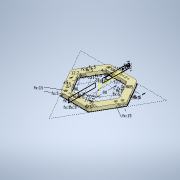
# Autodesk Inventor part: upper_board_mount
Saved by Autodesk Inventor 2021 (Build 250183000, 183)
## iProperties
Created: 2021-01-25
Part Number: upper_board_mount
Material: PC/ABS 플라스틱
Document SubType Name: Modeling
Designer: leejun
Density: 0.357273 g/cm^3
Appearance: 매끄러움 - 물푸레나무색
Author: leejun
Autodesk Inventor part; units mm, degrees
ref_plane "YZ Plane" through (0, 0, 0) normal (1, 0, 0) x (0, 1, 0)
ref_plane "XZ Plane" through (0, 0, 0) normal (0, 1, 0) x (-1, 0, 0)
ref_plane "XY Plane" through (0, 0, 0) normal (0, 0, 1) x (1, 0, 0)
sketch "스케치1" plane through (0, 0, 0) normal (0, 1, 0) x (-1, 0, 0)
  line L0 (128.6603, -74.282) -> (42.8868, -74.282) construction
  line L1 (-128.6603, -74.282) -> (0, 148.5641) construction
  line L2 (0, 148.5641) -> (128.6603, -74.282) construction
  line L3 (40, -69.282) -> (-40, -69.282) construction
  line L4 (-40, -69.282) -> (-40, -56.582) construction
  line L5 (-40, -56.582) -> (40, -56.582) construction
  line L6 (40, -56.582) -> (40, -69.282) construction
  line L7 (-80, 0) -> (-40, 69.282) construction
  line L8 (-40, 69.282) -> (-29.0015, 62.932) construction
  line L9 (-29.0015, 62.932) -> (-69.0015, -6.35) construction
  line L10 (-69.0015, -6.35) -> (-80, 0) construction
  line L11 (40, 69.282) -> (29.0015, 62.932) construction
  line L12 (29.0015, 62.932) -> (69.0015, -6.35) construction
  line L13 (69.0015, -6.35) -> (80, 0) construction
  line L14 (80, 0) -> (40, 69.282) construction
  line L15 (85.7735, 0) -> (42.8868, -74.282) construction
  line L16 (-42.8868, -74.282) -> (-85.7735, 0) construction
  line L17 (42.8868, 74.282) -> (-42.8868, 74.282) construction
  circle A0 centre (72.0007, 1.1551) radius 6.35 construction
  circle A1 centre (64.5007, 14.1455) radius 6.35 construction
  circle A2 centre (-35, -62.932) radius 6.35 construction
  circle A3 centre (-20, -62.932) radius 6.35 construction
  circle A4 centre (-37.0007, 61.7769) radius 6.35 construction
  circle A5 centre (-44.5007, 48.7865) radius 6.35 construction
  circle A6 centre (72.0007, 1.1551) radius 2.65 construction
  circle A7 centre (64.5007, 14.1455) radius 2.65 construction
  circle A8 centre (-20, -62.932) radius 2.65 construction
  circle A9 centre (-35, -62.932) radius 2.65 construction
  circle A10 centre (-44.5007, 48.7865) radius 2.65 construction
  circle A11 centre (-37.0007, 61.7769) radius 2.65 construction
  line L18 (40, -56.582) -> (-40, -69.282) construction
  line L19 (-40, -56.582) -> (40, -69.282) construction
  line L20 (69.0015, -6.35) -> (40, 69.282) construction
  line L21 (80, 0) -> (29.0015, 62.932) construction
  line L22 (-29.0015, 62.932) -> (-80, 0) construction
  line L23 (-69.0015, -6.35) -> (-40, 69.282) construction
  line L24 (72.0007, 1.1551) -> (64.5007, 14.1455) construction
  line L25 (-20, -62.932) -> (-35, -62.932) construction
  line L26 (-37.0007, 61.7769) -> (-44.5007, 48.7865) construction
  circle A12 centre (35, -62.932) radius 2.15
  circle A13 centre (20, -62.932) radius 2.15
  circle A14 centre (44.5007, 48.7865) radius 2.15
  circle A15 centre (37.0007, 61.7769) radius 2.15
  circle A16 centre (-72.0007, 1.1551) radius 2.15
  circle A17 centre (-64.5007, 14.1455) radius 2.15
  line L27 (42.8868, -74.282) -> (-42.8868, -74.282) construction
  line L28 (-42.8868, -74.282) -> (-128.6603, -74.282) construction
  line L29 (0, -62.932) -> (-54.5007, 31.466) construction
  line L30 (-54.5007, 31.466) -> (54.5007, 31.466) construction
  line L31 (54.5007, 31.466) -> (0, -62.932) construction
  line L32 (68.844, -27.6227) -> (58.344, -45.8093) construction
  line L33 (58.344, -45.8093) -> (40.1575, -35.3093) construction
  line L34 (40.1575, -35.3093) -> (50.6575, -17.1227) construction
  line L35 (50.6575, -17.1227) -> (68.844, -27.6227) construction
  line L36 (10.5, 73.432) -> (-10.5, 73.432) construction
  line L37 (-10.5, 73.432) -> (-10.5, 52.432) construction
  line L38 (-10.5, 52.432) -> (10.5, 52.432) construction
  line L39 (10.5, 52.432) -> (10.5, 73.432) construction
  line L40 (-58.344, -45.8093) -> (-68.844, -27.6227) construction
  line L41 (-68.844, -27.6227) -> (-50.6575, -17.1227) construction
  line L42 (-50.6575, -17.1227) -> (-40.1575, -35.3093) construction
  line L43 (-40.1575, -35.3093) -> (-58.344, -45.8093) construction
  line L44 (45.4075, -26.216) -> (-45.4075, -26.216) construction
  line L45 (-45.4075, -26.216) -> (0, 52.432) construction
  line L46 (0, 52.432) -> (45.4075, -26.216) construction
  line L47 (61.8712, 0) -> (30.9356, -53.582)
  line L48 (30.9356, -53.582) -> (-30.9356, -53.582)
  line L49 (-30.9356, -53.582) -> (-61.8712, 0)
  line L50 (-61.8712, 0) -> (-30.9356, 53.582)
  line L51 (-30.9356, 53.582) -> (30.9356, 53.582)
  line L52 (30.9356, 53.582) -> (61.8712, 0)
  line L53 (83.4641, 0) -> (41.7321, -72.282)
  line L54 (41.7321, -72.282) -> (-41.7321, -72.282)
  line L55 (-41.7321, -72.282) -> (-83.4641, 0)
  line L56 (-83.4641, 0) -> (-41.7321, 72.282)
  line L57 (-41.7321, 72.282) -> (41.7321, 72.282)
  line L58 (41.7321, 72.282) -> (83.4641, 0)
  line L59 (68.844, -27.6227) -> (40.1575, -35.3093) construction
  line L60 (58.344, -45.8093) -> (50.6575, -17.1227) construction
  circle A18 centre (54.5007, -31.466) radius 9.35 construction
  line L61 (71.0668, -21.4727) -> (73.9536, -26.4727) construction
  line L62 (73.9536, -26.4727) -> (59.9029, -50.8093) construction
  line L63 (59.9029, -50.8093) -> (54.1293, -50.8093) construction
  line L64 (54.8721, -12.1227) -> (49.0986, -12.1227) construction
  line L65 (49.0986, -12.1227) -> (35.0479, -36.4593) construction
  line L66 (35.0479, -36.4593) -> (37.9347, -41.4593) construction
  line L67 (16.9375, 53.582) -> (14.0507, 48.582) construction
  line L68 (14.0507, 48.582) -> (-14.0507, 48.582) construction
  line L69 (-14.0507, 48.582) -> (-16.9375, 53.582) construction
  line L70 (16.9375, 72.282) -> (14.0507, 77.282) construction
  line L71 (14.0507, 77.282) -> (-14.0507, 77.282) construction
  line L72 (-14.0507, 77.282) -> (-16.9375, 72.282) construction
  line L73 (-37.9347, -41.4593) -> (-35.0479, -36.4593) construction
  line L74 (-35.0479, -36.4593) -> (-49.0986, -12.1227) construction
  line L75 (-49.0986, -12.1227) -> (-54.8721, -12.1227) construction
  line L76 (-71.0668, -21.4727) -> (-73.9536, -26.4727) construction
  line L77 (-73.9536, -26.4727) -> (-59.9029, -50.8093) construction
  line L78 (-59.9029, -50.8093) -> (-54.1293, -50.8093) construction
  line L79 (42.8868, 74.282) -> (40, 69.282) construction
  line L80 (80, 0) -> (85.7735, 0) construction
  line L81 (0, 40) -> (-12.7, 40) construction
  line L82 (-12.7, 40) -> (-12.7, 52.7) construction
  line L83 (-12.7, 52.7) -> (0, 52.7) construction
  line L84 (0, 52.7) -> (0, 40) construction
  line L85 (12.7, -40) -> (0, -40) construction
  line L86 (0, -52.7) -> (12.7, -52.7) construction
  line L87 (12.7, -52.7) -> (12.7, -40) construction
  line L88 (12.7, -52.7) -> (-12.7, 52.7) construction
  line L89 (0, -40) -> (0, -52.7) construction
  line L90 (0, 52.7) -> (0, -52.7) construction
  line L91 (-12.7, 40) -> (-22.7, 40)
  line L92 (-22.7, 40) -> (-22.7, 53.582)
  line L93 (-22.7, 53.582) -> (-12.7, 53.582)
  line L94 (-12.7, 53.582) -> (-12.7, 40)
  line L95 (12.7, -40) -> (22.7, -40)
  line L96 (22.7, -40) -> (22.7, -53.582)
  line L97 (22.7, -53.582) -> (12.7, -53.582)
  line L98 (12.7, -53.582) -> (12.7, -40)
  line L99 (-12.7, 52.7) -> (-22.7, 52.7)
  line L100 (12.7, -52.7) -> (22.7, -52.7)
  point P0 (0, 0)
  point P1 (0, 0)
  point P2 (0, 0)
  point P3 (0, 0)
  point P4 (0, 0)
  point P5 (0, 0)
  point P6 (0, 0)
  dimension "d1" = 12.7
  dimension "d12" = 80
  dimension "d13" = 5.3
  dimension "d14" = 5
  dimension "d15" = 20
  dimension "d16" = 5
  dimension "d17" = 20
  dimension "d18" = 5
  dimension "d19" = 20
  dimension "d79" = 4.3
  dimension "d80" = 5
  dimension "d81" = 15
  dimension "d82" = 5
  dimension "d83" = 15
  dimension "d84" = 5
  dimension "d85" = 15
  dimension "d86" = 5
  dimension "d88" = 21
  dimension "d89" = 3
  dimension "d90" = 3
  dimension "d92" = 5
  dimension "d93" = 5
  dimension "d95" = 5
  dimension "d96" = 5
  dimension "d97" = 5
  dimension "d98" = 5
  dimension "d99" = 5
  dimension "d100" = 5
  dimension "d101" = 5
  dimension "d102" = 5
  dimension "d103" = 5
  dimension "d104" = 5
  dimension "d105" = 5
  dimension "d106" = 5
  dimension "d107" = 5
  dimension "d108" = 5
  dimension "d136" = 5
  dimension "d137" = 5
  dimension "d140" = 12.7
  dimension "d142" = 80
  dimension "d143" = 10
  constraints: 202 end point, 48 parallel, 28 point on line, 19 centre point, 16 equal length, 15 horizontal, 14 tangent, 12 coincident, 11 perpendicular, 10 equal radius, 9 midpoint, 2 collinear, 47 other
  measures "d1" distance of L12.end L13.end
  measures "d12" distance of L11.end L12.end
  measures "d13" diameter of A6
  measures "d14" distance from line of L13 A0.centre
  measures "d15" distance from line of A1.centre L13
  measures "d16" distance from line of L4 A2.centre
  measures "d17" distance from line of L4 A3.centre
  measures "d18" distance from line of L8 A4.centre
  measures "d19" distance from line of L8 A5.centre
  measures "d79" diameter of A12
  measures "d80" distance from line of A12.centre L6
  measures "d81" distance of A13.centre A12.centre
  measures "d82" distance from line of L11 A15.centre
  measures "d83" distance of A15.centre A14.centre
  measures "d84" distance from line of A16.centre L10
  measures "d85" distance of A17.centre A16.centre
  measures "d86" distance between parallel lines of L14 L2
  measures "d88" distance of L33.end L34.end
  measures "d89" distance between parallel lines of L14 L58
  measures "d90" distance between parallel lines of L12 L52
  measures "d92" distance from line of L32.start L61
  measures "d93" distance from line of L63 L32.end
  measures "d95" distance from line of L66 L33.end
  measures "d96" distance from line of L64 L34.end
  measures "d97" distance between parallel lines of L71 L57
  measures "d98" distance from line of L36.start L70
  measures "d99" distance from line of L72 L36.end
  measures "d100" distance between parallel lines of L51 L68
  measures "d101" distance from line of L38.end L67
  measures "d102" distance from line of L37.end L69
  measures "d103" distance between parallel lines of L49 L74
  measures "d104" distance from line of L42.end L73
  measures "d105" distance from line of L75 L41.end
  measures "d106" distance between parallel lines of L77 L55
  measures "d107" distance from line of L40.start L78
  measures "d108" distance from line of L76 L40.end
  measures "d136" distance between parallel lines of L53 L62
  measures "d137" distance between parallel lines of L65 L47
  measures "d140" distance of L85.end L86.start
  measures "d142" distance between parallel lines of L81 L85
  measures "d143" distance of L81.end L91.end
extrude "돌출18" add sketch "스케치1" along normal blind 10
sketch "스케치15" plane through (0, 0, 0) normal (0, -1, 0) x (1, 0, 0)
  line L0 (-41.7321, 72.282) -> (41.7321, 72.282) projected
  line L1 (-83.4641, 0) -> (-41.7321, 72.282) projected
  line L2 (-41.7321, -72.282) -> (-83.4641, 0) projected
  line L3 (41.7321, -72.282) -> (-41.7321, -72.282) projected
  line L4 (83.4641, 0) -> (41.7321, -72.282) projected
  line L5 (41.7321, 72.282) -> (83.4641, 0) projected
  circle A0 centre (-35, -62.932) radius 2.15 projected
  circle A1 centre (-20, -62.932) radius 2.15 projected
  circle A2 centre (-37.0007, 61.7769) radius 2.15 projected
  circle A3 centre (64.5007, 14.1455) radius 2.15 projected
  circle A4 centre (72.0007, 1.1551) radius 2.15 projected
  circle A5 centre (-44.5007, 48.7865) radius 2.15 projected
  line L6 (-61.8712, 0) -> (-30.9356, -53.582) projected
  line L7 (-30.9356, 53.582) -> (-61.8712, 0) projected
  line L8 (30.9356, 53.582) -> (-30.9356, 53.582) projected
  line L9 (61.8712, 0) -> (30.9356, 53.582) projected
  line L10 (30.9356, -53.582) -> (61.8712, 0) projected
  line L11 (-30.9356, -53.582) -> (30.9356, -53.582) projected
  line L12 (-44.5007, 48.7865) -> (-37.0007, 61.7769) construction
  line L13 (-40.1706, 46.2865) -> (-32.6706, 59.2769)
  line L14 (-41.3309, 64.2769) -> (-48.8309, 51.2865)
  arc A6 (-48.8309, 51.2865) -> (-40.1706, 46.2865) centre (-44.5007, 48.7865) ccw
  arc A7 (-32.6706, 59.2769) -> (-41.3309, 64.2769) centre (-37.0007, 61.7769) ccw
  line L15 (-35, -62.932) -> (-20, -62.932) construction
  line L16 (-35, -67.932) -> (-20, -67.932)
  line L17 (-20, -57.932) -> (-35, -57.932)
  arc A8 (-35, -57.932) -> (-35, -67.932) centre (-35, -62.932) ccw
  arc A9 (-20, -67.932) -> (-20, -57.932) centre (-20, -62.932) ccw
  circle A10 centre (72.0007, 1.1551) radius 2.15 projected
  circle A11 centre (64.5007, 14.1455) radius 2.15 projected
  line L18 (72.0007, 1.1551) -> (64.5007, 14.1455) construction
  line L19 (76.3309, 3.6551) -> (68.8309, 16.6455)
  line L20 (60.1706, 11.6455) -> (67.6706, -1.3449)
  arc A12 (67.6706, -1.3449) -> (76.3309, 3.6551) centre (72.0007, 1.1551) ccw
  arc A13 (68.8309, 16.6455) -> (60.1706, 11.6455) centre (64.5007, 14.1455) ccw
  point P0 (0, 0)
  point P1 (-40.7507, 55.2817)
  point P2 (-27.5, -62.932)
  point P3 (68.2507, 7.6503)
  dimension "d148" = 5
  constraints: 24 end point, 12 point on circle, 12 tangent, 6 centre point, 3 midpoint, 3 parallel, 2 equal radius, 1 horizontal
  measures "d148" radius of A6
extrude "돌출20" add sketch "스케치15" along normal blind 5 contours A6 L14 A7 L13 | A8 L17 A9 L16 | A12 L20 A13 L19
fillet "모깎기4" radius 10 12 edges at (41.7321, 5, 72.282) (83.4641, 5, 0) (41.7321, 5, -72.282) (-41.7321, 5, -72.282) (-83.4641, 5, 0) (-41.7321, 5, 72.282) (-61.8712, 5, 0) (-30.9356, 5, 53.582) (30.9356, 5, 53.582) (61.8712, 5, 0) (30.9356, 5, -53.582) (-30.9356, 5, -53.582)
fillet "모깎기4" radius 3 12 edges at (62.0007, 0, 18.4756) (72.5809, 0, 10.1503) (74.5007, 0, -3.175) (63.9206, 0, 5.1503) (-47.0007, 0, 44.4564) (-45.0809, 0, 57.7817) (-34.5007, 0, 66.107) (-36.4206, 0, 52.7817) (-27.5, 0, -57.932) (-15, 0, -62.932) (-27.5, 0, -67.932) (-40, 0, -62.932)
sketch "스케치18" plane through (0, 10, 0) normal (0, 1, 0) x (1, 0, 0)
  arc A0 (-44.6188, -67.282) -> (-35.9585, -72.282) centre (-35.9585, -62.282) ccw projected
  line L0 (-35.9585, -72.282) -> (35.9585, -72.282) projected
  arc A1 (35.9585, -72.282) -> (44.6188, -67.282) centre (35.9585, -62.282) ccw projected
  line L1 (44.6188, -67.282) -> (80.5774, -5) projected
  arc A2 (80.5774, -5) -> (80.5774, 5) centre (71.9171, 0) ccw projected
  line L2 (80.5774, 5) -> (44.6188, 67.282) projected
  arc A3 (44.6188, 67.282) -> (35.9585, 72.282) centre (35.9585, 62.282) ccw projected
  line L3 (35.9585, 72.282) -> (-35.9585, 72.282) projected
  arc A4 (-35.9585, 72.282) -> (-44.6188, 67.282) centre (-35.9585, 62.282) ccw projected
  line L4 (-44.6188, 67.282) -> (-80.5774, 5) projected
  arc A5 (-80.5774, 5) -> (-80.5774, -5) centre (-71.9171, 0) ccw projected
  line L5 (-80.5774, -5) -> (-44.6188, -67.282) projected
  circle A6 centre (-35, 62.932) radius 2.15 projected
  circle A7 centre (-20, 62.932) radius 2.15 projected
  circle A8 centre (-37.0007, -61.7769) radius 2.15 projected
  circle A9 centre (64.5007, -14.1455) radius 2.15 projected
  circle A10 centre (72.0007, -1.1551) radius 2.15 projected
  circle A11 centre (-44.5007, -48.7865) radius 2.15 projected
  line L6 (-58.9845, 5) -> (-33.8224, 48.582) projected
  arc A12 (-25.1621, 53.582) -> (-33.8224, 48.582) centre (-25.1621, 43.582) ccw projected
  line L7 (-25.1621, 53.582) -> (25.1621, 53.582) projected
  arc A13 (33.8224, 48.582) -> (25.1621, 53.582) centre (25.1621, 43.582) ccw projected
  line L8 (33.8224, 48.582) -> (58.9845, 5) projected
  arc A14 (58.9845, -5) -> (58.9845, 5) centre (50.3242, 0) ccw projected
  line L9 (58.9845, -5) -> (33.8224, -48.582) projected
  arc A15 (25.1621, -53.582) -> (33.8224, -48.582) centre (25.1621, -43.582) ccw projected
  line L10 (25.1621, -53.582) -> (-25.1621, -53.582) projected
  arc A16 (-33.8224, -48.582) -> (-25.1621, -53.582) centre (-25.1621, -43.582) ccw projected
  line L11 (-33.8224, -48.582) -> (-58.9845, -5) projected
  arc A17 (-58.9845, 5) -> (-58.9845, -5) centre (-50.3242, 0) ccw projected
  circle A18 centre (-35, 62.932) radius 3.9
  circle A19 centre (-20, 62.932) radius 3.9
  point P0 (0, 0)
  dimension "d167" = 7.8
  constraints: 2 centre point, 2 coincident, 1 equal radius
  measures "d167" diameter of A18
extrude "돌출23" cut sketch "스케치18" against normal blind 3 contours A18 | A19
pattern_circular "원형 패턴5" count 3 over 360 about axis through (0, -10, 0) along (0, 1, 0) of "돌출23"
sketch "스케치25" plane through (0, 0, 0) normal (1, 0, 0) x (0, 1, 0)
  line L0 (12, -91) -> (24.7, -91)
  line L1 (24.7, -91) -> (24.7, -11)
  line L2 (24.7, -11) -> (12, -11)
  line L3 (12, -11) -> (12, -91)
  line L4 (12, 11) -> (24.7, 11)
  line L5 (24.7, 11) -> (24.7, 91)
  line L6 (24.7, 91) -> (12, 91)
  line L7 (12, 91) -> (12, 11)
  line L8 (-4.94, 0) -> (29.64, 0) projected
  line L9 (10, -67.282) -> (10, -5) projected
  circle A0 centre (18.35, -86) radius 6.35
  circle A1 centre (18.35, -86) radius 2.6
  circle A2 centre (18.35, -71) radius 2.6
  point P0 (0, 0)
  dimension "d210" = 12.7
  dimension "d211" = 80
  dimension "d212" = 22
  dimension "d213" = 2
  dimension "d214" = 5
  dimension "d215" = 15
  dimension "d216" = 5.2
  constraints: 16 end point, 4 parallel, 3 centre point, 2 equal length, 2 horizontal, 2 perpendicular, 2 tangent, 1 coincident, 1 collinear, 1 equal radius, 1 vertical alignment, 1 other
  measures "d210" distance of L1.end L2.end
  measures "d211" distance of L0.end L1.end
  measures "d212" distance between parallel lines of L4 L2
  measures "d213" distance between parallel lines of L9 L3
  measures "d214" distance from line of L0 A1.centre
  measures "d215" distance of A2.centre A1.centre
  measures "d216" diameter of A1
sketch "스케치26" plane through (0, 10, 0) normal (0, 1, 0) x (1, 0, 0)
  circle A0 centre (64.5007, -14.1455) radius 3.9 projected
  circle A1 centre (72.0007, -1.1551) radius 3.9 projected
  circle A2 centre (-44.5007, -48.7865) radius 3.9 projected
  circle A3 centre (-37.0007, -61.7769) radius 3.9 projected
  circle A4 centre (-20, 62.932) radius 3.9 projected
  circle A5 centre (-35, 62.932) radius 3.9 projected
  arc A6 (-44.6188, -67.282) -> (-35.9585, -72.282) centre (-35.9585, -62.282) ccw projected
  line L0 (-35.9585, -72.282) -> (35.9585, -72.282) projected
  arc A7 (35.9585, -72.282) -> (44.6188, -67.282) centre (35.9585, -62.282) ccw projected
  line L1 (44.6188, -67.282) -> (80.5774, -5) projected
  arc A8 (80.5774, -5) -> (80.5774, 5) centre (71.9171, 0) ccw projected
  line L2 (80.5774, 5) -> (44.6188, 67.282) projected
  arc A9 (44.6188, 67.282) -> (35.9585, 72.282) centre (35.9585, 62.282) ccw projected
  line L3 (35.9585, 72.282) -> (-35.9585, 72.282) projected
  arc A10 (-35.9585, 72.282) -> (-44.6188, 67.282) centre (-35.9585, 62.282) ccw projected
  line L4 (-44.6188, 67.282) -> (-80.5774, 5) projected
  arc A11 (-80.5774, 5) -> (-80.5774, -5) centre (-71.9171, 0) ccw projected
  line L5 (-80.5774, -5) -> (-44.6188, -67.282) projected
  line L6 (-58.9845, 5) -> (-33.8224, 48.582) projected
  arc A12 (-25.1621, 53.582) -> (-33.8224, 48.582) centre (-25.1621, 43.582) ccw projected
  line L7 (-25.1621, 53.582) -> (25.1621, 53.582) projected
  arc A13 (33.8224, 48.582) -> (25.1621, 53.582) centre (25.1621, 43.582) ccw projected
  line L8 (33.8224, 48.582) -> (58.9845, 5) projected
  arc A14 (58.9845, -5) -> (58.9845, 5) centre (50.3242, 0) ccw projected
  line L9 (58.9845, -5) -> (33.8224, -48.582) projected
  arc A15 (25.1621, -53.582) -> (33.8224, -48.582) centre (25.1621, -43.582) ccw projected
  line L10 (25.1621, -53.582) -> (-25.1621, -53.582) projected
  arc A16 (-33.8224, -48.582) -> (-25.1621, -53.582) centre (-25.1621, -43.582) ccw projected
  line L11 (-33.8224, -48.582) -> (-58.9845, -5) projected
  arc A17 (-58.9845, 5) -> (-58.9845, -5) centre (-50.3242, 0) ccw projected
  line L12 (-25.1621, 53.582) -> (25.1621, 53.582) projected
  line L13 (35.9585, 72.282) -> (-35.9585, 72.282) projected
  line L14 (25.1621, 53.582) -> (0, 53.582)
  line L15 (0, 53.582) -> (0, 72.282)
  line L16 (0, 72.282) -> (25.1621, 72.282)
  line L17 (25.1621, -53.582) -> (-25.1621, -53.582) projected
  line L18 (-35.9585, -72.282) -> (35.9585, -72.282) projected
  line L19 (0, -53.582) -> (-25.1621, -53.582)
  line L20 (-25.1621, -72.282) -> (0, -72.282)
  line L21 (0, -72.282) -> (0, -53.582)
  circle A18 centre (25, 62.932) radius 2.1
  circle A19 centre (10, 62.932) radius 2.1
  circle A20 centre (25, 62.932) radius 9.35 construction
  circle A21 centre (-25, -62.932) radius 2.1
  circle A22 centre (-10, -62.932) radius 2.1
  circle A23 centre (-25, -62.932) radius 9.35 construction
  line L22 (0, 129.02) -> (0, -127.67) projected
  point P0 (0, 0)
  dimension "d217" = 4.2
  dimension "d225" = 15
  dimension "d226" = 15
  dimension "d227" = 10
  dimension "d228" = 10
  constraints: 12 end point, 6 centre point, 4 tangent, 3 equal radius, 3 parallel, 2 coincident, 2 horizontal, 2 horizontal alignment, 2 midpoint, 1 perpendicular, 1 point on line
  measures "d217" diameter of A18
  measures "d225" distance of A21.centre A22.centre
  measures "d226" distance of A19.centre A18.centre
  measures "d227" distance from line of L22 A22.centre
  measures "d228" distance from line of L22 A19.centre
extrude "돌출30" cut sketch "스케치26" against normal through all contours A18 | A19 | A21 | A22
sketch "스케치27" plane through (0, 0, 0) normal (0, -1, 0) x (1, 0, 0)
  circle A0 centre (25, -62.932) radius 2.1 projected
  circle A1 centre (10, -62.932) radius 2.1 projected
  circle A2 centre (-10, 62.932) radius 2.1 projected
  circle A3 centre (-25, 62.932) radius 2.1 projected
  line L0 (-10, 58.7751) -> (-13.6, 60.8536)
  line L1 (-13.6, 60.8536) -> (-13.6, 65.0105)
  line L2 (-13.6, 65.0105) -> (-10, 67.089)
  line L3 (-10, 67.089) -> (-6.4, 65.0105)
  line L4 (-6.4, 65.0105) -> (-6.4, 60.8536)
  line L5 (-6.4, 60.8536) -> (-10, 58.7751)
  circle A4 centre (-25, 62.932) radius 2.1 projected
  line L6 (-25, 58.7751) -> (-28.6, 60.8536)
  line L7 (-28.6, 60.8536) -> (-28.6, 65.0105)
  line L8 (-28.6, 65.0105) -> (-25, 67.089)
  line L9 (-25, 67.089) -> (-21.4, 65.0105)
  line L10 (-21.4, 65.0105) -> (-21.4, 60.8536)
  line L11 (-21.4, 60.8536) -> (-25, 58.7751)
  line L12 (25, -67.089) -> (21.4, -65.0105)
  line L13 (21.4, -65.0105) -> (21.4, -60.8536)
  line L14 (21.4, -60.8536) -> (25, -58.7751)
  line L15 (25, -58.7751) -> (28.6, -60.8536)
  line L16 (28.6, -60.8536) -> (28.6, -65.0105)
  line L17 (28.6, -65.0105) -> (25, -67.089)
  line L18 (10, -67.089) -> (6.4, -65.0105)
  line L19 (6.4, -65.0105) -> (6.4, -60.8536)
  line L20 (6.4, -60.8536) -> (10, -58.7751)
  line L21 (10, -58.7751) -> (13.6, -60.8536)
  line L22 (13.6, -60.8536) -> (13.6, -65.0105)
  line L23 (13.6, -65.0105) -> (10, -67.089)
  point P0 (0, 0)
  dimension "d222" = 7.2
  constraints: 48 end point, 4 coincident, 4 vertical, 3 parallel, 52 other
  measures "d222" distance between parallel lines of L1 L4
extrude "돌출31" cut sketch "스케치27" against normal blind 2 contours A0 | A1 | L0 L1 L2 L3 L4 L5 | L6 L7 L8 L9 L10 L11 | L12 L13 L14 L15 L16 L17 | L18 L19 L20 L21 L22 L23
sketch "스케치28" plane through (0, 10, 0) normal (0, 1, 0) x (1, 0, 0)
  circle A0 centre (-10, -62.932) radius 2.1 projected
  circle A1 centre (10, 62.932) radius 2.1 projected
  circle A2 centre (-25, -62.932) radius 2.1 projected
  circle A3 centre (25, 62.932) radius 2.1 projected
  circle A4 centre (64.5007, -14.1455) radius 3.9 projected
  circle A5 centre (72.0007, -1.1551) radius 3.9 projected
  circle A6 centre (-44.5007, -48.7865) radius 3.9 projected
  circle A7 centre (-37.0007, -61.7769) radius 3.9 projected
  circle A8 centre (-20, 62.932) radius 3.9 projected
  circle A9 centre (-35, 62.932) radius 3.9 projected
  arc A10 (-44.6188, -67.282) -> (-35.9585, -72.282) centre (-35.9585, -62.282) ccw projected
  line L0 (-35.9585, -72.282) -> (35.9585, -72.282) projected
  arc A11 (35.9585, -72.282) -> (44.6188, -67.282) centre (35.9585, -62.282) ccw projected
  line L1 (44.6188, -67.282) -> (80.5774, -5) projected
  arc A12 (80.5774, -5) -> (80.5774, 5) centre (71.9171, 0) ccw projected
  line L2 (80.5774, 5) -> (44.6188, 67.282) projected
  arc A13 (44.6188, 67.282) -> (35.9585, 72.282) centre (35.9585, 62.282) ccw projected
  line L3 (35.9585, 72.282) -> (-35.9585, 72.282) projected
  arc A14 (-35.9585, 72.282) -> (-44.6188, 67.282) centre (-35.9585, 62.282) ccw projected
  line L4 (-44.6188, 67.282) -> (-80.5774, 5) projected
  arc A15 (-80.5774, 5) -> (-80.5774, -5) centre (-71.9171, 0) ccw projected
  line L5 (-80.5774, -5) -> (-44.6188, -67.282) projected
  line L6 (-58.9845, 5) -> (-33.8224, 48.582) projected
  arc A16 (-25.1621, 53.582) -> (-33.8224, 48.582) centre (-25.1621, 43.582) ccw projected
  line L7 (-25.1621, 53.582) -> (25.1621, 53.582) projected
  arc A17 (33.8224, 48.582) -> (25.1621, 53.582) centre (25.1621, 43.582) ccw projected
  line L8 (33.8224, 48.582) -> (58.9845, 5) projected
  arc A18 (58.9845, -5) -> (58.9845, 5) centre (50.3242, 0) ccw projected
  line L9 (58.9845, -5) -> (33.8224, -48.582) projected
  arc A19 (25.1621, -53.582) -> (33.8224, -48.582) centre (25.1621, -43.582) ccw projected
  line L10 (25.1621, -53.582) -> (-25.1621, -53.582) projected
  arc A20 (-33.8224, -48.582) -> (-25.1621, -53.582) centre (-25.1621, -43.582) ccw projected
  line L11 (-33.8224, -48.582) -> (-58.9845, -5) projected
  arc A21 (-58.9845, 5) -> (-58.9845, -5) centre (-50.3242, 0) ccw projected
  line L12 (2, 66.432) -> (5, 66.432)
  line L13 (5, 66.432) -> (5, 59.432)
  line L14 (5, 59.432) -> (2, 59.432)
  line L15 (2, 59.432) -> (2, 66.432)
  line L16 (2, 66.432) -> (5, 59.432) construction
  line L17 (5, 66.432) -> (2, 59.432) construction
  line L18 (16, 66.432) -> (19, 66.432)
  line L19 (19, 66.432) -> (19, 59.432)
  line L20 (19, 59.432) -> (16, 59.432)
  line L21 (16, 59.432) -> (16, 66.432)
  line L22 (16, 66.432) -> (19, 59.432) construction
  line L23 (19, 66.432) -> (16, 59.432) construction
  line L24 (-19, -59.432) -> (-16, -59.432)
  line L25 (-16, -59.432) -> (-16, -66.432)
  line L26 (-16, -66.432) -> (-19, -66.432)
  line L27 (-19, -66.432) -> (-19, -59.432)
  line L28 (-19, -59.432) -> (-16, -66.432) construction
  line L29 (-16, -59.432) -> (-19, -66.432) construction
  line L30 (-5, -59.432) -> (-2, -59.432)
  line L31 (-2, -59.432) -> (-2, -66.432)
  line L32 (-2, -66.432) -> (-5, -66.432)
  line L33 (-5, -66.432) -> (-5, -59.432)
  line L34 (-5, -59.432) -> (-2, -66.432) construction
  line L35 (-2, -59.432) -> (-5, -66.432) construction
  line L36 (0, 129.02) -> (0, -127.67) projected
  point P0 (0, 0)
  point P1 (3.5, 62.932)
  point P2 (17.5, 62.932)
  point P3 (-17.5, -62.932)
  point P4 (-3.5, -62.932)
  point P5 (-3.5, -62.932)
  point P6 (3.5, 62.932)
  point P7 (17.5, 62.932)
  point P8 (-17.5, -62.932)
  dimension "d229" = 3
  dimension "d230" = 7
  dimension "d231" = 7.5
  dimension "d234" = 2
  constraints: 48 end point, 12 midpoint, 8 parallel, 5 equal length, 4 horizontal, 4 horizontal alignment, 4 perpendicular, 1 point on line, 2 other
  measures "d229" distance of L31.end L32.end
  measures "d230" distance of L12.end L13.end
  measures "d231" distance of A1.centre point (17.5, 62.932)
  measures "d234" distance between parallel lines of L36 L15
extrude "돌출32" cut sketch "스케치28" against normal through all contours L12 L13 L14 L15 | L18 L19 L20 L21 | L24 L25 L26 L27 | L30 L31 L32 L33
equation "\"d16\" = d14"
equation "\"d17\" = d15"
equation "\"d18\" = d14"
equation "\"d19\" = d15"
